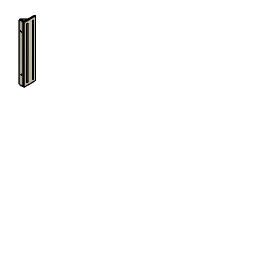
Mounting Left (Autodesk Fusion 360 design; units mm, degrees)
Autodesk Fusion 360 part; units mm, degrees
sketch "Sketch1" plane through (0, 18.2563, 0) normal (0, 1, 0) x (-1, 0, 0)
  line L0 (428.571, 352.5901) -> (428.571, 293.5351)
  line L1 (428.571, 293.5351) -> (479.3844, 293.5351)
  arc A0 (492.0844, 280.8351) -> (479.3844, 293.5351) centre (479.3844, 280.8351) ccw
  line L2 (492.0844, 280.8351) -> (492.0844, 170.3924)
  arc A1 (479.3844, 157.6924) -> (492.0844, 170.3924) centre (479.3844, 170.3924) ccw
  line L3 (479.3844, 157.6924) -> (379.1345, 157.6924)
  arc A2 (366.4345, 170.3924) -> (379.1345, 157.6924) centre (379.1345, 170.3924) ccw
  line L4 (366.4345, 170.3924) -> (366.4345, 365.2901)
  line L5 (366.4345, 365.2901) -> (415.871, 365.2901)
  arc A3 (428.571, 352.5901) -> (415.871, 365.2901) centre (415.871, 352.5901) ccw
  line L6 (472.0327, 153.7035) -> (472.0327, 110.5235)
  line L7 (472.0327, 110.5235) -> (272.8342, 110.5235)
  line L8 (272.8342, 110.5235) -> (272.8342, 153.7035)
  line L9 (272.8342, 153.7035) -> (472.0327, 153.7035)
  line L10 (357.5015, 303.1464) -> (352.4754, 303.1464)
  arc A4 (352.4754, 303.1464) -> (349.9354, 300.6064) centre (352.4754, 300.6064) ccw
  line L11 (349.9354, 300.6064) -> (349.9353, 294.0949)
  arc A5 (349.9353, 294.0949) -> (352.4753, 291.5549) centre (352.4753, 294.0949) ccw
  line L12 (352.4753, 291.5549) -> (357.5015, 291.5549)
  arc A6 (360.0415, 289.0149) -> (357.5015, 291.5549) centre (357.5015, 289.0149) ccw
  line L13 (360.0415, 289.0149) -> (360.0415, 224.7549)
  line L14 (343.1642, 207.8775) -> (284.3089, 207.8775)
  arc A7 (281.7689, 210.4175) -> (284.3089, 207.8775) centre (284.3089, 210.4175) ccw
  line L15 (281.7689, 210.4175) -> (281.7689, 213.7509)
  arc A8 (281.7689, 213.7509) -> (279.2289, 216.2909) centre (279.2289, 213.7509) ccw
  line L16 (279.2289, 216.2909) -> (269.7942, 216.2909)
  arc A9 (269.7942, 216.2909) -> (267.2542, 213.7509) centre (269.7942, 213.7509) ccw
  line L17 (267.2542, 213.7509) -> (267.2542, 209.8586)
  arc A10 (264.7142, 207.3186) -> (267.2542, 209.8586) centre (264.7142, 209.8586) ccw
  line L18 (264.7142, 207.3186) -> (195.981, 207.3186)
  arc A11 (193.441, 209.8586) -> (195.981, 207.3186) centre (195.981, 209.8586) ccw
  line L19 (193.441, 209.8586) -> (193.441, 212.2563)
  arc A12 (193.441, 212.2563) -> (191.0274, 214.6699) centre (191.0274, 212.2563) ccw
  line L20 (191.0274, 214.6699) -> (184.0403, 214.6699)
  arc A13 (184.0403, 214.6699) -> (182.1012, 212.7308) centre (184.0403, 212.7308) ccw
  line L21 (182.1012, 212.7308) -> (182.1012, 201.4539)
  arc A14 (182.1012, 201.4539) -> (182.7112, 200.8439) centre (182.7112, 201.4539) ccw
  line L22 (182.7112, 200.8439) -> (182.9015, 200.8439)
  arc A15 (183.5115, 200.2339) -> (182.9015, 200.8439) centre (182.9015, 200.2339) ccw
  line L23 (183.5115, 200.2339) -> (183.5115, 121.5175)
  arc A16 (170.8115, 108.8175) -> (183.5115, 121.5175) centre (170.8115, 121.5175) ccw
  line L24 (170.8115, 108.8175) -> (21.7935, 108.8175)
  arc A17 (9.0935, 121.5175) -> (21.7935, 108.8175) centre (21.7935, 121.5175) ccw
  line L25 (9.0935, 121.5175) -> (9.0935, 382.5281)
  line L26 (9.0935, 382.5281) -> (4.9467, 382.5281)
  line L27 (4.9467, 382.5281) -> (4.9467, 408.8477)
  arc A18 (360.0415, 379.6488) -> (347.4641, 392.3482) centre (347.3415, 379.6488) ccw
  line L28 (360.0415, 379.6488) -> (360.0415, 305.6864)
  arc A19 (357.5015, 303.1464) -> (360.0415, 305.6864) centre (357.5015, 305.6864) ccw
  line L29 (418.6909, 72.6852) -> (471.3254, 72.6852)
  line L30 (471.3254, 72.6852) -> (471.3254, 15.5352)
  line L31 (471.3254, 15.5352) -> (418.6909, 15.5352)
  arc A20 (412.3409, 9.1852) -> (418.6909, 15.5352) centre (412.3409, 15.5352) ccw
  line L32 (412.3409, 9.1852) -> (241.5223, 9.1852)
  arc A21 (177.9281, 15.5352) -> (184.2781, 9.1852) centre (184.2781, 15.5352) ccw
  line L33 (177.9281, 15.5352) -> (177.9281, 79.0484)
  arc A22 (184.2781, 85.3984) -> (177.9281, 79.0484) centre (184.2781, 79.0484) ccw
  line L34 (184.2781, 85.3984) -> (225.0204, 85.3984)
  line L35 (225.0204, 85.3984) -> (225.0204, 77.837)
  line L36 (225.0204, 77.837) -> (241.7413, 77.837)
  line L37 (241.7413, 77.837) -> (241.9712, 96.6279)
  line L38 (241.9712, 96.6279) -> (412.3409, 96.6279)
  arc A23 (418.6909, 90.2779) -> (412.3409, 96.6279) centre (412.3409, 90.2779) ccw
  line L39 (418.6909, 90.2779) -> (418.6909, 72.6852)
  line L40 (-4.42, 194.5895) -> (9.0935, 194.5895)
  line L41 (9.0935, 194.5895) -> (9.0935, -108.98)
  line L42 (9.0935, -108.98) -> (-4.42, -108.98)
  line L43 (-4.42, -108.98) -> (-4.42, 194.5895)
  line L44 (-1.42, 194.5895) -> (-1.42, -108.98)
  line L45 (9.0935, 179.3281) -> (-1.42, 179.3281)
  line L46 (360.0415, 224.7549) -> (354.6743, 213.2448)
  line L47 (354.6743, 213.2448) -> (343.1642, 207.8775)
  circle A24 centre (207.7084, 193.413) radius 2.159
  line L48 (3.8368, 179.3281) -> (3.8368, -108.98) construction
  circle A25 centre (3.8368, -58.98) radius 1.5875
  circle A26 centre (3.8368, 16.02) radius 1.5875
  circle A27 centre (3.8368, 169.5895) radius 1.5875
  line L49 (-290.0096, 92.5057) -> (-290.0096, 7.234)
  line L50 (-290.0096, 7.234) -> (-465.075, 7.234)
  line L51 (-465.075, 7.234) -> (-465.075, 92.5057)
  line L52 (-4.42, 42.8048) -> (49.4042, 42.8048)
  line L53 (9.0935, 118.6971) -> (75.9448, 118.6971) construction
  circle A28 centre (3.8368, 67.8048) radius 1.5875
  line L54 (-500, 143.9311) -> (-500, 126.9933)
  arc A29 (-500, 143.9311) -> (-500, 126.9933) centre (-509.464, 135.4622) ccw
  line L55 (-500, 79.9338) -> (-500, 0)
  line L56 (-500, 0) -> (-107.8843, 0)
  spline S0 degree 3 poles (-107.8843, 0) (-106.6495, 0.0607) (-105.4498, -0.1313) (-102.6874, -1.0161) (-101.1244, -1.8659) (-96.1633, -5.2179) (-92.725, -8.5214) (-86.2474, -13.8936) (-83.361, -16.033) (-78.6115, -18.3434) (-76.9814, -18.9534) (-73.5162, -19.796) (-71.7498, -20) (-69.9424, -20) knots 0 0 0 0 0.370897 0.370897 0.871374 0.871374 1.959694 1.959694 2.776333 2.776333 3.183727 3.183727 3.602468 3.602468 3.602468 3.602468
  line L57 (-69.9424, -20) -> (69.9424, -20)
  spline S1 degree 3 poles (69.9424, -20) (73.0012, -20) (75.8629, -19.4155) (81.7994, -16.9675) (84.6203, -15.0806) (91.091, -10.0169) (94.5926, -6.6002) (99.7197, -2.7488) (101.3808, -1.6813) (103.8464, -0.6268) (104.658, -0.3574) (106.2841, -0.0279) (107.079, 0.0396) (107.8843, 0) knots 0 0 0 0 0.917641 0.917641 1.92675 1.92675 3.392474 3.392474 4.093018 4.093018 4.419465 4.419465 4.727908 4.727908 4.727908 4.727908
  line L58 (107.8843, 0) -> (500, 0)
  line L59 (500, 0) -> (500, 79.9338)
  line L60 (500, 79.9338) -> (522.3504, 79.9338)
  line L61 (522.3504, 79.9338) -> (522.3504, 105.4918)
  line L62 (522.3504, 105.4918) -> (526.6736, 105.4918)
  line L63 (526.6736, 105.4918) -> (526.6736, 224.0816)
  line L64 (526.6736, 224.0816) -> (520.32, 224.0816)
  line L65 (520.32, 224.0816) -> (520.32, 294.692)
  line L66 (520.32, 294.692) -> (520.32, 294.703)
  spline S2 degree 3 poles (172.9706, 440.32) (272.7886, 440.32) (347.139, 432.8584) (431.6124, 406.7549) (455.5556, 394.5767) (490.0751, 366.2568) (500.0952, 352.6411) (509.9527, 335.0646) (514.0209, 326.6095) (518.829, 309.9549) (520.32, 302.5094) (520.32, 294.703) knots 0 0 0 0 29.945399 29.945399 46.557158 46.557158 60.60518 60.60518 68.217831 68.217831 73.312075 73.312075 73.312075 73.312075
  line L67 (172.9706, 440.32) -> (-172.9706, 440.32)
  spline S3 degree 3 poles (-520.32, 294.703) (-520.32, 303.749) (-518.2237, 312.6579) (-513.118, 328.5698) (-507.4943, 341.8443) (-483.2112, 373.9486) (-466.3523, 386.2242) (-428.6068, 408.1818) (-399.6888, 418.1178) (-315.5941, 435.6039) (-252.1803, 440.32) (-172.9706, 440.32) knots 0 0 0 0 2.71381 2.71381 6.253873 6.253873 10.935243 10.935243 18.75486 18.75486 30.231285 30.231285 30.231285 30.231285
  line L68 (-520.32, 294.703) -> (-520.32, 294.692)
  line L69 (-520.32, 294.692) -> (-520.32, 232.0032)
  line L70 (-520.32, 232.0032) -> (-520.3202, 224.0815)
  line L71 (-520.3202, 224.0815) -> (-525.7287, 224.0816)
  line L72 (-525.7287, 224.0816) -> (-525.7316, 110.9551)
  line L73 (-525.7316, 110.9551) -> (-520.7141, 110.955)
  line L74 (-520.7141, 110.955) -> (-520.7148, 79.9338)
  line L75 (-520.7148, 79.9338) -> (-500, 79.9338)
  line L76 (500, 126.268) -> (500, 153.0045)
  arc A30 (500, 126.268) -> (500, 153.0045) centre (508.5619, 139.6363) ccw
  line L77 (-500, 228.2042) -> (-500, 232.0142)
  arc A31 (-500, 228.2042) -> (-500, 232.0142) centre (-500, 230.1092) ccw
  arc A32 (500, 232.0142) -> (500, 228.2042) centre (500, 230.1092) ccw
  line L78 (500, 232.0142) -> (500, 228.2042)
  circle A33 centre (512.0079, 186.5029) radius 10.795
  circle A34 centre (-511.1752, 213.2838) radius 3.81
  circle A35 centre (-511.1752, 162.4838) radius 3.81
  circle A36 centre (-511.1752, 105.3338) radius 3.81
  circle A37 centre (511.1752, 213.2838) radius 3.81
  circle A38 centre (511.1752, 162.4838) radius 3.81
  circle A39 centre (511.1752, 105.3338) radius 3.81
  arc A40 (233.164, 152.101) -> (226.836, 152.101) centre (230, 170.8864) ccw
  line L79 (4.9467, 408.8477) -> (82.7509, 408.8477)
  line L80 (82.7509, 408.8477) -> (82.7509, 386.4984)
  line L81 (82.7509, 386.4984) -> (103.5865, 386.4984)
  line L82 (103.5865, 386.4984) -> (103.5865, 405.762)
  line L83 (103.5865, 405.762) -> (119.5134, 405.762)
  line L84 (119.5134, 405.762) -> (119.5134, 411.2029)
  line L85 (119.5134, 411.2029) -> (212.7672, 411.2029)
  line L86 (212.7672, 411.2029) -> (212.7672, 392.3482)
  line L87 (212.7672, 392.3482) -> (347.4641, 392.3482)
  arc A41 (-226.836, 152.101) -> (-233.164, 152.101) centre (-230, 170.8864) ccw
  line L88 (-4.42, 398.8196) -> (-4.42, 95.25)
  line L89 (-4.42, 95.25) -> (-164.44, 95.25)
  line L90 (-164.44, 95.25) -> (-164.44, 398.8196)
  line L91 (-164.44, 398.8196) -> (-4.42, 398.8196)
  circle A42 centre (-177.1872, 297.5787) radius 2.159
  circle A43 centre (-214.6628, 193.5123) radius 2.159
  circle A44 centre (-388.1565, 393.2992) radius 2.159
  circle A45 centre (-282.2406, 407.3174) radius 2.159
  circle A46 centre (-493.5531, 297.8904) radius 2.159
  circle A47 centre (-408.3272, 101.9987) radius 2.159
  circle A48 centre (-473.8573, 131.3177) radius 2.159
  circle A49 centre (-324.5072, 101.9987) radius 2.159
  circle A50 centre (-239.4172, 101.9987) radius 2.159
  circle A51 centre (-398.1653, 131.3177) radius 2.159
  circle A52 centre (-244.6336, 193.9737) radius 2.159
  circle A53 centre (224.1328, 101.9987) radius 2.159
  circle A54 centre (5.6928, 204.8687) radius 2.159
  arc A55 (214.9811, 195.9051) -> (215.0468, 191.5876) centre (215.0138, 193.7463) ccw
  arc A56 (215.0468, 191.5876) -> (214.9811, 195.9051) centre (215.014, 193.7463) ccw
  arc A57 (215.0119, 150.1869) -> (215.0119, 145.8689) centre (215.0118, 148.0279) ccw
  arc A58 (215.0119, 145.8689) -> (215.0119, 150.1869) centre (215.012, 148.0279) ccw
  circle A59 centre (114.9128, 101.9987) radius 2.159
  circle A60 centre (89.5128, 411.8787) radius 2.159
  circle A61 centre (5.6928, 101.9987) radius 2.159
  circle A62 centre (5.6928, 297.5787) radius 2.159
  circle A63 centre (5.6928, 411.8787) radius 2.159
  circle A64 centre (-491.999, 85.217) radius 2.159
  circle A65 centre (0.1314, 56.9243) radius 6.985
  circle A66 centre (58.04, 11.75) radius 4
  circle A67 centre (121.8609, 85.217) radius 2.159
  circle A68 centre (-270.7296, 34.5828) radius 2.54
  circle A69 centre (-29.2895, 11.4414) radius 2.54
  circle A70 centre (-154.8913, 70.6424) radius 1.905
  circle A71 centre (-154.8913, 19.8424) radius 1.905
  circle A72 centre (121.8609, 8.001) radius 2.159
  circle A73 centre (-57.289, 56.9243) radius 9.525
  circle A74 centre (-11.0854, 11.4414) radius 1.27
  circle A75 centre (-191.7213, 19.8424) radius 1.905
  circle A76 centre (-270.7296, 71.3118) radius 2.54
  circle A77 centre (58.04, 56.2) radius 4
  circle A78 centre (-47.4937, 11.4414) radius 1.27
  circle A79 centre (-191.7213, 70.6424) radius 1.905
  line L92 (-183.7415, 69.6959) -> (-171.4865, 69.6959)
  line L93 (-171.4865, 69.6959) -> (-171.4865, 66.0556)
  line L94 (-171.4865, 66.0556) -> (-154.9321, 66.0556)
  line L95 (-154.9321, 66.0556) -> (-154.9321, 27.0556)
  line L96 (-154.9321, 27.0556) -> (-176.0865, 27.0556)
  line L97 (-176.0865, 27.0556) -> (-176.0865, 23.2779)
  line L98 (-176.0865, 23.2779) -> (-183.7415, 23.2779)
  line L99 (-183.7415, 23.2779) -> (-183.7415, 29.4869)
  line L100 (-183.7415, 29.4869) -> (-190.7415, 29.4869)
  line L101 (-190.7415, 29.4869) -> (-190.7415, 63.4869)
  line L102 (-190.7415, 63.4869) -> (-183.7415, 63.4869)
  line L103 (-183.7415, 63.4869) -> (-183.7415, 69.6959)
  circle A80 centre (493.7399, 117.3795) radius 2.159
  circle A81 centre (-491.999, 8.001) radius 2.159
  circle A82 centre (369.6053, 398.877) radius 2.159
  circle A83 centre (366.3728, 101.9987) radius 2.159
  arc A84 (245.0207, 150.1853) -> (244.9517, 145.8678) centre (244.9863, 148.0266) ccw
  arc A85 (244.9517, 145.8678) -> (245.0207, 150.1853) centre (244.9862, 148.0266) ccw
  circle A86 centre (140.3586, 8.007) radius 2.159
  circle A87 centre (-177.1872, 101.9987) radius 2.159
  circle A88 centre (-224.1772, 101.9987) radius 2.159
  circle A89 centre (238.1028, 101.9987) radius 2.159
  circle A90 centre (478.5816, 334.3996) radius 2.159
  arc A91 (245.0211, 195.9038) -> (244.9554, 191.5863) centre (244.9883, 193.745) ccw
  arc A92 (244.9554, 191.5863) -> (245.0211, 195.9038) centre (244.9882, 193.745) ccw
  circle A93 centre (357.3764, 297.813) radius 2.159
  circle A94 centre (102.5905, 410.606) radius 2.159
  line L104 (-465.075, 92.5057) -> (-290.0096, 92.5057)
  circle A95 centre (357.3764, 210.6675) radius 2.159
  circle A96 centre (231.3193, 408.9455) radius 2.159
  circle A97 centre (274.4728, 210.6675) radius 2.159
  circle A98 centre (357.3764, 399.6405) radius 2.159
  circle A99 centre (475.0114, 144.9236) radius 2.159
  circle A100 centre (270.2874, 144.9236) radius 2.159
  circle A101 centre (270.2874, 119.2696) radius 2.159
  circle A102 centre (475.0114, 119.2696) radius 2.159
  circle A103 centre (425.25, 7.9753) radius 2.159
  circle A104 centre (234.0846, 85.223) radius 2.159
  circle A105 centre (464.366, 85.1913) radius 2.159
  circle A106 centre (425.25, 85.1913) radius 2.159
  circle A107 centre (464.366, 7.9753) radius 2.159
  circle A108 centre (186.0567, 210.6675) radius 2.159
  circle A109 centre (-245.3372, 148.2606) radius 2.159
  circle A110 centre (-493.5531, 115.0104) radius 2.159
  circle A111 centre (-177.1872, 178.1987) radius 2.159
  line L105 (-400.8755, 328.0702) -> (-424.3755, 328.0702)
  line L106 (-424.3755, 328.0702) -> (-424.3755, 353.8202)
  line L107 (-424.3755, 353.8202) -> (-400.8755, 353.8202)
  line L108 (-400.8755, 353.8202) -> (-400.8755, 328.0702)
  circle A112 centre (-175.2863, 409.9134) radius 2.159
  circle A113 centre (-177.1872, 162.9587) radius 2.159
  circle A114 centre (-215.3665, 147.7992) radius 2.159
  circle A115 centre (140.3586, 85.223) radius 2.159
  circle A116 centre (234.0846, 8.007) radius 2.159
  line L109 (241.5223, 9.1852) -> (241.5223, 12.9465)
  line L110 (241.5223, 12.9465) -> (223.6432, 12.9465)
  line L111 (223.6432, 12.9465) -> (223.6432, 9.1852)
  line L112 (223.6432, 9.1852) -> (184.2781, 9.1852)
  line L113 (-442.5639, 278.7168) -> (-442.5639, 326.4668)
  line L114 (-442.5639, 326.4668) -> (-381.5639, 326.4668)
  line L115 (-381.5639, 326.4668) -> (-381.5639, 278.7168)
  line L116 (-381.5639, 278.7168) -> (-442.5639, 278.7168)
  arc A117 (-233.175, 136.7885) -> (-226.825, 136.7885) centre (-230, 136.7885) ccw
  line L117 (-233.175, 136.7885) -> (-233.175, 151.8364)
  arc A118 (-233.164, 152.101) -> (-233.175, 151.8364) centre (-230, 151.8364) ccw
  arc A119 (-226.825, 151.8364) -> (-226.836, 152.101) centre (-230, 151.8364) ccw
  line L118 (-226.825, 151.8364) -> (-226.825, 136.7885)
  arc A120 (226.825, 136.7885) -> (233.175, 136.7885) centre (230, 136.7885) ccw
  line L119 (226.825, 136.7885) -> (226.825, 151.8364)
  arc A121 (226.836, 152.101) -> (226.825, 151.8364) centre (230, 151.8364) ccw
  arc A122 (233.175, 151.8364) -> (233.164, 152.101) centre (230, 151.8364) ccw
  line L120 (233.175, 151.8364) -> (233.175, 136.7885)
  dimension "d1" = 3
  dimension "d37" = 3.175
  dimension "d38" = 50
  dimension "d39" = 25
  dimension "d41" = 125
  dimension "d77" = 75.8924
  dimension "d78" = 151.7848
  constraint horizontal L40
  constraint vertical L41
  constraint horizontal L42
  constraint vertical L43
  constraint coincident L40 L44.start
  constraint coincident L42 L44.end
  constraint perpendicular L42 L44
  constraint coincident L44 L45.end
  constraint perpendicular L44 L45
  constraint midpoint L45 L48.start
  constraint coincident L42 L48.end
  constraint perpendicular L42 L48
  constraint coincident L48 A25.centre
  constraint coincident L48 A26.centre
  constraint coincident L48 A27.centre
  constraint equal A25 A26
  constraint midpoint L43 L52.start
  constraint perpendicular L44 L52
  constraint coincident L41 L53.start
  constraint coincident L25 L53.start
  constraint perpendicular L41 L53
  constraint symmetric A27 L53 A28
  measures "d1" distance of L43 L44
  measures "d37" diameter of A25
  measures "d38" distance of L42 A25.centre
  measures "d39" distance of L40 A27.centre
  measures "d41" distance of L48.end A26.centre
  measures "d77" distance of L40.end L53.start
  measures "d78" distance of L40 L52
extrude "Extrude1" add sketch "Sketch1" along normal blind 3 contours L25 L40 L41 L44 L45 | L25 L41 L44 L45 L52 A65 | L44 A65 | A61 makes body 1
extrude "Extrude2" add sketch "Sketch1" along normal blind 31.2437 separate body contours L40 L43 L44 L88 A65 | L43 L44 A65 | L43 L44 L52 A65 makes body 2
sketch "Sketch2" plane through (0, 21.2563, 0) normal (0, 1, 0) x (-1, 0, 0)
  line L0 (9.0935, 42.8048) -> (9.0935, 194.5895)
  line L1 (-1.42, 194.5895) -> (-1.42, 42.8048)
  line L2 (-1.42, 189.5895) -> (9.0935, 189.5895)
  line L3 (9.0935, 189.5895) -> (9.0935, 194.5895)
  line L4 (9.0935, 194.5895) -> (-1.42, 194.5895)
  line L5 (-1.42, 194.5895) -> (-1.42, 189.5895)
  line L6 (-1.42, 189.5895) -> (9.0935, 194.5895) construction
  line L7 (9.0935, 189.5895) -> (-1.42, 194.5895) construction
  line L8 (-1.42, 42.8048) -> (9.0935, 42.8048)
  line L9 (9.0935, 42.8048) -> (9.0935, 47.8048)
  line L10 (9.0935, 47.8048) -> (-1.42, 47.8048)
  line L11 (-1.42, 47.8048) -> (-1.42, 42.8048)
  line L12 (-1.42, 42.8048) -> (9.0935, 47.8048) construction
  line L13 (9.0935, 42.8048) -> (-1.42, 47.8048) construction
  circle A0 centre (3.8368, 169.5895) radius 1.5875
  line L14 (-1.42, -48.98) -> (9.0935, -48.98)
  line L15 (9.0935, -48.98) -> (9.0935, -68.98)
  line L16 (9.0935, -68.98) -> (-1.42, -68.98)
  line L17 (-1.42, -68.98) -> (-1.42, -48.98)
  line L18 (-1.42, -48.98) -> (9.0935, -68.98) construction
  line L19 (9.0935, -48.98) -> (-1.42, -68.98) construction
  line L20 (9.0935, 194.5895) -> (-1.42, 194.5895)
  line L21 (-1.42, 42.8048) -> (9.0935, 42.8048)
  circle A1 centre (3.8368, 67.8048) radius 1.5875
  circle A2 centre (3.8368, 67.8048) radius 3
  circle A3 centre (3.8368, 169.5895) radius 3
  line L22 (9.0935, 194.5895) -> (-1.42, 194.5895)
  point P0 (3.8368, 192.0895)
  point P1 (3.8368, 45.3048)
  point P2 (3.8368, -58.98)
  dimension "d12" = 5
  dimension "d13" = 5
  dimension "d43" = 20
  dimension "d81" = 6
  constraint horizontal L2
  constraint perpendicular L2 L3
  constraint parallel L2 L4
  constraint parallel L3 L5
  constraint coincident L1 L2.start
  constraint coincident L6 P0
  constraint coincident L7 P0
  constraint horizontal L8
  constraint perpendicular L8 L9
  constraint parallel L8 L10
  constraint parallel L9 L11
  constraint coincident L12 P1
  constraint coincident L13 P1
  constraint horizontal L14
  constraint perpendicular L14 L15
  constraint parallel L14 L16
  constraint parallel L15 L17
  constraint coincident L1 L14.start
  constraint coincident L18 P2
  constraint coincident L19 P2
  constraint concentric A1 A2
  constraint concentric A0 A3
  constraint equal A2 A3
  constraint coincident L0.end L3.end
  constraint coincident L0 L9.end
  measures "d12" distance of L0.start L9.end
  measures "d13" distance of L2.end L0.end
  measures "d43" distance of L14.end L15.end
  measures "d81" diameter of A3
sketch "Sketch4" plane through (4.42, 0, 0) normal (1, 0, 0) x (0, 1, 0)
  line L0 (18.2563, 194.5895) -> (18.2563, 42.8048)
  line L1 (18.2563, 42.8048) -> (49.5, 42.8048)
  line L2 (49.5, 42.8048) -> (49.5, 194.5895)
  line L3 (49.5, 194.5895) -> (18.2563, 194.5895)
  line L4 (42, 187.0895) -> (42, 50.3048) construction
  line L5 (43.55, 50.3048) -> (43.55, 187.0895)
  arc A0 (28.55, 187.0895) -> (25.45, 187.0895) centre (27, 187.0895) ccw
  line L6 (40.45, 187.0895) -> (40.45, 50.3048)
  line L7 (25.45, 187.0895) -> (25.45, 50.3048)
  line L8 (28.55, 50.3048) -> (28.55, 187.0895)
  arc A1 (43.55, 187.0895) -> (40.45, 187.0895) centre (42, 187.0895) ccw
  arc A2 (40.45, 50.3048) -> (43.55, 50.3048) centre (42, 50.3048) ccw
  arc A3 (25.45, 50.3048) -> (28.55, 50.3048) centre (27, 50.3048) ccw
  line L9 (18.2563, 194.5895) -> (-3, 194.5895)
  line L10 (-3, 194.5895) -> (-3, 42.8048)
  line L11 (-3, 42.8048) -> (18.2562, 42.8048)
  line L12 (18.2563, 42.8048) -> (18.2563, 194.5895)
  dimension "d89" = 15
  dimension "d90" = 0
  dimension "d91" = 3.1
  dimension "d93" = 15
  dimension "d97" = 7.5
  dimension "d98" = 7.5
  dimension "d99" = 21.2563
  dimension "d103" = 30
  constraint tangent L6 A2
  constraint tangent L5 A2
  constraint parallel L5 L6
  constraint tangent L5 A1
  constraint tangent L6 A1
  constraint horizontal L9
  constraint vertical L10
  constraint horizontal L11
  constraint vertical L12
  constraint coincident L0.start L3.end
  measures "d91" diameter of A2
  measures "d93" distance of A3.centre L4.end
  measures "d97" distance of L3 L4.start
  measures "d98" distance of L1 L4.end
  measures "d99" distance of L0.start L9.end
  measures "d103" distance of A0.centre L10
extrude "Extrude4" cut sketch "Sketch4" along normal through all and the other way through all contours L5 L6 A1 A2 | A0 L7 L8 A3 bodies 2
extrude "Extrude3" add sketch "Sketch2" along normal blind 10 separate body contours L0 L1 L8 L9 L10 L11 L21 | L0 L1 L2 L3 L4 L5 L20 L22 makes body 3 at (-2.0845, 24.5896, 42.8048) makes body 4 at (-2.0845, 24.5896, 189.5895)
chamfer "Chamfer1" distance 10 distance2 10 2 edges at (-9.0935, 31.2563, 192.0895) (-9.0935, 31.2563, 45.3048) measured on face at (-2.0845, 31.2563, 191.2562) measured on face at (-2.0845, 31.2563, 44.4714) on bodies 3 4
equation "d4 = 52.5 mm - PlyAndAcrylicThick"
equation "d33 = 0.0 °"
equation "d37 = 1 / 8 * 1\""
equation "d77 = d78 / 2"
equation "d98 = d97"
equation "d99 = PlyAndAcrylicThick"
equation "PlyAndAcrylicThick = ( 23 / 32 * 1\" ) + ( 3 mm )"
named bodies: "Panel Part", "Rack Part", "Lower Chamfer", "Upper Chamfer"
